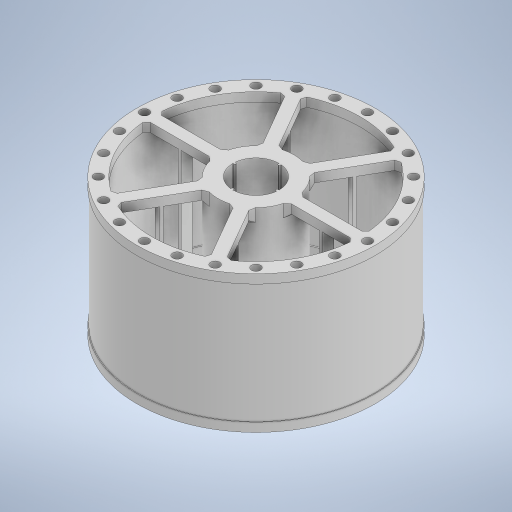
# Autodesk Inventor part: WheelV1Printable
Saved by Autodesk Inventor 2024.2 (Build 282272000, 272)
## iProperties
Created: 2024-01-02
Part Number: WheelV1Printable
Material: Generisch
Document SubType Name: Modeling
Designer: chris
Density: 1 g/cm^3
Appearance: Vorgabe
Author: chris
Autodesk Inventor part; units mm, degrees
ref_plane "YZ Plane" through (0, 0, 0) normal (1, 0, 0) x (0, 1, 0)
ref_plane "XZ Plane" through (0, 0, 0) normal (0, 1, 0) x (-1, 0, 0)
ref_plane "XY Plane" through (0, 0, 0) normal (0, 0, 1) x (1, 0, 0)
sketch "Skizze1" plane through (0, 0, 0) normal (0, 0, 1) x (1, 0, 0)
  circle A0 centre (0, 0) radius 7.75
  circle A1 centre (0, 0) radius 12.75
  dimension "d2" = 15.5
  dimension "d3" = 25.5
  constraints: 2 centre point, 1 coincident
  measures "d2" diameter of A0
  measures "d3" diameter of A1
extrude "Extrusion1" add sketch "Skizze1" along normal mid plane 46.2
sketch "Skizze3" plane through (0, 0, 23.1) normal (0, 0, 1) x (1, 0, 0)
  circle A0 centre (0, 0) radius 35
  circle A1 centre (0, 0) radius 40
  dimension "d6" = 70
  dimension "d7" = 80
  constraints: 2 centre point, 2 coincident
  measures "d6" diameter of A0
  measures "d7" diameter of A1
extrude "Extrusion2" add sketch "Skizze3" against normal blind 3
sketch "Skizze4" plane through (0, 0, 23.1) normal (0, 0, 1) x (1, 0, 0)
  circle A0 centre (0, 0) radius 12.75 construction
  circle A1 centre (0, 0) radius 35 construction
  line L0 (-12.7499, 0.05) -> (-35, 0.05)
  line L1 (-12.7499, 0.05) -> (-12.4499, 0.05) construction
  arc A2 (-12.7499, 0.05) -> (-12.7, 1.1281) centre (0, 0) ccw
  arc A3 (-35, 0.05) -> (-34.9637, 1.5937) centre (0, 0) ccw
  line L2 (-12.6, -1.95) -> (-34.9456, -1.95)
  dimension "d13" = 0.3
  dimension "d21" = 2
  constraints: 10 point on circle, 6 end point, 3 horizontal, 2 centre point, 2 concentric
  measures "d13" distance of L0.start L1.end
  measures "d21" distance between parallel lines of L0 L2
extrude "Extrusion4" add sketch "Skizze4" against normal blind 3
chamfer "Fasen1" distance 1.25 angle 45 2 edges at (-12.6, -1.95, 21.6) (-34.9456, -1.95, 21.6)
mirror "Spiegeln2" about plane through (0, 0, 0) normal (0, 1, 0) of "Extrusion4", "Fasen1"
pattern_circular "Runde Anordnung2" count 6 over 360 about axis through (0, 0, -10) along (0, 0, 1) of "Extrusion4", "Fasen1", "Spiegeln2"
chamfer "Fasen2" distance 1.25 angle 45 7 edges at (6.375, 11.0418, 20.1) (12.6492, -1.5999, 20.1) (12.6492, 1.5999, 20.1) (-6.375, 11.0418, 20.1) (6.375, -11.0418, 20.1) (-6.375, -11.0418, 20.1) (-12.75, 0, 20.1)
sketch "Skizze5" plane through (0, 0, 23.1) normal (0, 0, 1) x (1, 0, 0)
  circle A0 centre (0, 0) radius 40 construction
  line L0 (0, -40) -> (0, -35) construction
  arc A1 (-14.6585, -31.7825) -> (14.6585, -31.7825) centre (0, 0) ccw construction
  circle A2 centre (0, -37.5) radius 1.5
  dimension "d33" = 3
  constraints: 2 end point, 1 centre point, 1 midpoint, 1 point on circle, 1 vertical, 1 vertical alignment, 1 other
  measures "d33" diameter of A2
extrude "Extrusion5" cut sketch "Skizze5" against normal blind 3
pattern_circular "Runde Anordnung3" count 24 over 360 about axis through (0, 0, -10) along (0, 0, 1) of "Extrusion5"
mirror "Spiegeln3" about plane through (0, 0, 0) normal (0, 0, 1) of "Extrusion4", "Fasen1", "Spiegeln2", "Runde Anordnung2", "Extrusion2", "Extrusion5", "Runde Anordnung3", "Fasen2"
sketch "Skizze6" plane through (0, 0, 0) normal (0, 0, 1) x (1, 0, 0)
  circle A0 centre (0, 0) radius 7.75 projected
  line L0 (0, 7.75) -> (0, 7.12)
  line L1 (0, 7.12) -> (0.75, 7.12)
  line L2 (0.75, 7.12) -> (0.75, 7.7136)
  arc A1 (0.75, 7.7136) -> (1.464, 7.6105) centre (0, 0) ccw
  dimension "d39" = 0.63
  dimension "d40" = 0.75
  constraints: 6 end point, 6 point on circle, 2 vertical, 1 centre point, 1 concentric, 1 perpendicular
  measures "d39" distance of L0.start L0.end
  measures "d40" distance of L0.end L1.end
extrude "Extrusion6" add sketch "Skizze6" along normal mid plane 46.2 contours A0 L2 L1 L0 picked at (0.4168, 7.3246)
pattern_circular "Runde Anordnung4" count 4 over 360 about axis through (0, 0, -10) along (0, 0, 1) of "Extrusion6"
fillet "Rundung1" radius 0.35 8 edges at (0.75, 7.12, 0) (0, 7.12, 0) (-7.12, 0, 0) (-7.12, 0.75, 0) (-0.75, -7.12, 0) (0, -7.12, 0) (7.12, 0, 0) (7.12, -0.75, 0)
sketch "Skizze7" plane through (0, 0, 0) normal (0, 0, 1) x (1, 0, 0)
  circle A0 centre (0, 0) radius 39.75
  circle A1 centre (0, 0) radius 39.25
  circle A2 centre (0, 0) radius 35.4
  circle A3 centre (0, 0) radius 35.9
  dimension "d47" = 79.5
  dimension "d48" = 78.5
  dimension "d51" = 70.8
  dimension "d52" = 71.8
  constraints: 4 centre point, 4 coincident
  measures "d47" diameter of A0
  measures "d48" diameter of A1
  measures "d51" diameter of A2
  measures "d52" diameter of A3
extrude "Extrusion7" add sketch "Skizze7" along normal mid plane 40.2
sketch "Skizze8" plane through (0, 0, 0) normal (0, 0, 1) x (1, 0, 0)
  line L0 (15.1591, -30.1563) -> (5.2363, -12.9695) projected
  line L1 (10.1977, -21.5629) -> (13.5752, -19.6129)
  line L2 (18.5366, -28.2063) -> (8.6137, -11.0195) projected
  line L3 (13.5752, -19.6129) -> (13.8252, -20.0459)
  line L4 (13.8252, -20.0459) -> (10.4477, -21.9959)
  line L5 (10.4477, -21.9959) -> (9.9477, -21.1299)
  line L6 (9.9477, -21.1299) -> (13.3252, -19.1799)
  line L7 (13.3252, -19.1799) -> (13.5752, -19.6129)
  point P0 (0, 0)
  dimension "d53" = 0.5
  dimension "d54" = 1
  constraints: 12 end point, 4 point on line, 2 midpoint, 2 perpendicular
  measures "d53" distance of L1.end L3.end
  measures "d54" distance of L4.end L5.end
extrude "Extrusion8" add sketch "Skizze8" along normal mid plane 40.2
pattern_circular "Runde Anordnung5" count 6 over 360 about axis through (0, 0, -10) along (0, 0, 1) of "Extrusion8"
